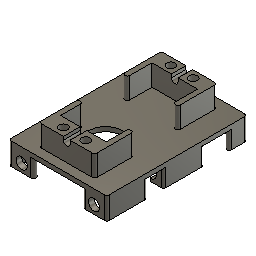
ServoMount (Autodesk Fusion 360 design; units mm, degrees)
Autodesk Fusion 360 part; units mm, degrees
note: some values were not read from the file. Set by a fixed rule: which sketch regions a step uses.
sketch "Base" plane through (0, 0, 0) normal (0, 1, 0) x (1, 0, 0)
  line L0 (0, 0) -> (44, 0)
  line L1 (44, 0) -> (44, 63)
  line L2 (44, 63) -> (0, 63)
  line L3 (0, 63) -> (0, 0)
  dimension "d1" = 44
  dimension "d2" = 63
  constraint horizontal L0
  constraint vertical L1
  constraint horizontal L2
  constraint vertical L3
  constraint coincident L0.start L3.end
  measures "d1" distance of L0.start L0.end
  measures "d2" distance of L0.start L2.end
extrude "Extrude1" add sketch "Base" along normal blind 2
sketch "Servo_Mount" plane through (0, 2, 0) normal (0, 1, 0) x (-1, 0, 0)
  line L0 (0, -63) -> (0, 0)
  line L1 (0, 0) -> (-44, 0)
  line L2 (-44, 0) -> (-44, -63)
  line L3 (-44, -63) -> (0, -63)
  line L4 (-10.75, -59) -> (-33.25, -59)
  line L5 (-33.25, -4) -> (-10.75, -4)
  line L6 (-9.5, -52.5) -> (-34.5, -52.5)
  line L7 (-9.5, -11.5) -> (-34.5, -11.5)
  line L8 (-22, 0) -> (-22, -72)
  circle A0 centre (-17, -55.75) radius 1.875
  circle A1 centre (-27, -55.75) radius 1.875
  circle A2 centre (-17, -7.5) radius 1.875
  circle A3 centre (-27, -7.5) radius 1.875
  circle A4 centre (-22, -21.5) radius 7.5
  arc A5 (-9.5, -5.25) -> (-10.75, -4) centre (-10.75, -5.25) ccw
  arc A6 (-33.25, -4) -> (-34.5, -5.25) centre (-33.25, -5.25) ccw
  arc A7 (-10.75, -59) -> (-9.5, -57.75) centre (-10.75, -57.75) ccw
  arc A8 (-34.5, -57.75) -> (-33.25, -59) centre (-33.25, -57.75) ccw
  line L9 (-11.75, -52.5) -> (-11.75, -42.625)
  line L10 (-11.75, -20.375) -> (-11.75, -11.5)
  line L11 (-9.5, -5.25) -> (-9.5, -20.375)
  line L12 (-9.5, -42.625) -> (-9.5, -57.75)
  line L13 (-32.25, -52.5) -> (-32.25, -42.625)
  line L14 (-32.25, -20.375) -> (-32.25, -11.5)
  line L15 (-34.5, -57.75) -> (-34.5, -42.625)
  line L16 (-34.5, -20.375) -> (-34.5, -5.25)
  arc A9 (-10.625, -41.5) -> (-11.75, -42.625) centre (-10.625, -42.625) ccw
  arc A10 (-9.5, -42.625) -> (-10.625, -41.5) centre (-10.625, -42.625) ccw
  arc A11 (-32.25, -42.625) -> (-33.375, -41.5) centre (-33.375, -42.625) ccw
  arc A12 (-33.375, -41.5) -> (-34.5, -42.625) centre (-33.375, -42.625) ccw
  arc A13 (-33.375, -21.5) -> (-32.25, -20.375) centre (-33.375, -20.375) ccw
  arc A14 (-34.5, -20.375) -> (-33.375, -21.5) centre (-33.375, -20.375) ccw
  arc A15 (-10.625, -21.5) -> (-9.5, -20.375) centre (-10.625, -20.375) ccw
  arc A16 (-11.75, -20.375) -> (-10.625, -21.5) centre (-10.625, -20.375) ccw
  circle A17 centre (-27, -7.5) radius 2.875
  circle A18 centre (-17, -7.5) radius 2.875
  circle A19 centre (-27, -55.75) radius 2.875
  circle A20 centre (-17, -55.75) radius 2.875
  point P0 (-9.5, -59)
  point P1 (-34.5, -59)
  point P2 (-9.5, -4)
  dimension "d5" = 25
  dimension "d6" = 55
  dimension "d7" = 4
  dimension "d8" = 9.5
  dimension "d9" = 25
  dimension "d10" = 6.5
  dimension "d11" = 7.5
  dimension "d12" = 41
  dimension "d13" = 41
  dimension "d14" = 2.25
  dimension "d15" = 2.25
  dimension "d16" = 3.75
  dimension "d17" = 3.75
  dimension "d18" = 3.25
  dimension "d19" = 3.25
  dimension "d20" = 5
  dimension "d21" = 5
  dimension "d22" = 3.75
  dimension "d23" = 3.75
  dimension "d24" = 4
  dimension "d25" = 4
  dimension "d26" = 5
  dimension "d27" = 5
  dimension "d28" = 15
  dimension "d29" = 10
  dimension "d34" = 1.25
  dimension "d35" = 1.25
  dimension "d36" = 1.25
  dimension "d37" = 1.25
  dimension "d38" = 1.125
  dimension "d39" = 1.125
  dimension "d40" = 1.125
  dimension "d41" = 1.125
  dimension "d42" = 1.125
  dimension "d43" = 1.125
  dimension "d44" = 1.125
  dimension "d45" = 1.125
  dimension "d57" = 22.25
  dimension "d119" = 5.75
  dimension "d120" = 5.75
  dimension "d121" = 5.75
  dimension "d122" = 5.75
  constraint horizontal L4
  constraint vertical L15
  constraint horizontal L5
  constraint vertical L11
  constraint coincident L6.start L11
  constraint perpendicular L6 L15
  constraint coincident L7.start L11
  constraint coincident L7.end L15
  constraint perpendicular L7 L15
  constraint coincident L6 L9.start
  constraint perpendicular L7 L9
  constraint coincident L6 L13.start
  constraint perpendicular L6 L13
  constraint midpoint L1 L8.start
  constraint perpendicular L3 L8
  constraint coincident L8 A4.centre
  constraint coincident P2 L5
  constraint coincident P2 L11
  constraint tangent L5 A5
  constraint tangent A5 L11
  constraint tangent L5 A6
  constraint tangent A6 L15
  constraint coincident P0 L4
  constraint coincident P0 L11
  constraint tangent L4 A7
  constraint tangent A7 L11
  constraint coincident P1 L15
  constraint coincident P1 L4
  constraint tangent A8 L15
  constraint tangent L4 A8
  constraint collinear L9 L10
  constraint collinear L11 L12
  constraint collinear L13 L14
  constraint collinear L15 L16
  constraint tangent L9 A9
  constraint tangent L12 A10
  constraint coincident A9.start A10.end
  constraint tangent L13 A11
  constraint tangent L15 A12
  constraint coincident A11.end A12.start
  constraint tangent L14 A13
  constraint tangent L16 A14
  constraint coincident A13.start A14.end
  constraint tangent L11 A15
  constraint tangent L10 A16
  constraint coincident A15.start A16.end
  constraint concentric A3 A17
  constraint concentric A2 A18
  constraint concentric A1 A19
  constraint concentric A0 A20
  measures "d5" distance of P0 P1
  measures "d6" distance of P0 P2
  measures "d7" distance of L3 L4
  measures "d8" distance of L0 L11
  measures "d9" distance of L6.start L6.end
  measures "d10" distance of L4 L6
  measures "d11" distance of L5 L7
  measures "d12" distance of L9.start L10.end
  measures "d13" distance of L13.start L14.end
  measures "d14" distance of L9 L11
  measures "d15" distance of L13 L15
  measures "d16" diameter of A0
  measures "d17" diameter of A1
  measures "d18" distance of L4 A0.centre
  measures "d19" distance of L4 A1.centre
  measures "d20" distance of L8 A1.centre
  measures "d21" distance of L8 A0.centre
  measures "d22" diameter of A2
  measures "d23" diameter of A3
  measures "d24" distance of L7 A3.centre
  measures "d25" distance of L7 A2.centre
  measures "d26" distance of L8 A2.centre
  measures "d27" distance of L8 A3.centre
  measures "d28" diameter of A4
  measures "d29" distance of L7 A4.centre
  measures "d34" radius of A5
  measures "d35" radius of A6
  measures "d36" radius of A7
  measures "d37" radius of A8
  measures "d38" radius of A9
  measures "d39" radius of A10
  measures "d40" radius of A11
  measures "d41" radius of A12
  measures "d42" radius of A13
  measures "d43" radius of A14
  measures "d44" radius of A15
  measures "d45" radius of A16
  measures "d57" distance of A9.centre A15.centre
  measures "d119" diameter of A17
  measures "d120" diameter of A18
  measures "d121" diameter of A19
  measures "d122" diameter of A20
extrude "Extrude2" cut sketch "Servo_Mount" against normal blind 9 contours L8 A4 | L8 A4
extrude "Extrude3" add sketch "Servo_Mount" along normal blind 9.5 contours L4 L6 L8 A7 L12 | L4 L6 L8 A8 L15 | L5 L7 L8 A6 L16 | L5 L7 L8 A5 L11 | L6 L9 L12 A9 A10 | L6 L13 L15 A11 A12 | L7 L10 L11 A15 A16 | L7 L14 L16 A13 A14 | A17 | A18 | A19 | A20
sketch "Top_Through_Front" plane through (0, 0, -4) normal (0, 0, 1) x (1, 0, 0)
  line L0 (10.75, 2) -> (33.25, 2)
  line L1 (33.25, 2) -> (33.25, 11.5)
  line L2 (33.25, 11.5) -> (10.75, 11.5)
  line L3 (10.75, 11.5) -> (10.75, 2)
  line L4 (20.5, 11.5) -> (23.5, 11.5)
  line L5 (23.5, 11.5) -> (23.5, 10)
  line L6 (20.5, 10) -> (20.5, 11.5)
  arc A0 (20.5, 10) -> (22, 8.5) centre (22, 10) ccw
  arc A1 (22, 8.5) -> (23.5, 10) centre (22, 10) ccw
  point P0 (20.5, 8.5)
  dimension "d50" = 3
  dimension "d51" = 3
  dimension "d52" = 9.75
  dimension "d53" = 1.5
  dimension "d54" = 1.5
  constraint horizontal L4
  constraint vertical L5
  constraint vertical L6
  constraint coincident L2 L4.start
  constraint coincident P0 L6
  constraint tangent L6 A0
  constraint tangent L5 A1
  constraint coincident A0.end A1.start
  measures "d50" distance of L4.start L4.end
  measures "d51" distance of L4.start P0
  measures "d52" distance of L1 L5
  measures "d53" radius of A0
  measures "d54" radius of A1
extrude "Extrude4" cut sketch "Top_Through_Front" against normal blind 15 contours L2 L4 L5 L6 A0 A1
sketch "Top_Through_Back" plane through (0, 0, -59) normal (0, 0, -1) x (-1, 0, 0)
  line L0 (-33.25, 2) -> (-10.75, 2)
  line L1 (-10.75, 2) -> (-10.75, 11.5)
  line L2 (-10.75, 11.5) -> (-33.25, 11.5)
  line L3 (-33.25, 11.5) -> (-33.25, 2)
  line L4 (-23.5, 11.5) -> (-20.5, 11.5)
  line L5 (-20.5, 11.5) -> (-20.5, 10)
  line L6 (-23.5, 10) -> (-23.5, 11.5)
  arc A0 (-22, 8.5) -> (-20.5, 10) centre (-22, 10) ccw
  arc A1 (-23.5, 10) -> (-22, 8.5) centre (-22, 10) ccw
  point P0 (-23.5, 8.5)
  dimension "d58" = 3
  dimension "d59" = 3
  dimension "d60" = 9.75
  dimension "d61" = 1.5
  dimension "d62" = 1.5
  constraint horizontal L4
  constraint vertical L5
  constraint vertical L6
  constraint coincident L2 L4.start
  constraint tangent L5 A0
  constraint coincident P0 L6
  constraint tangent L6 A1
  constraint coincident A0.start A1.end
  measures "d58" distance of L4.start L4.end
  measures "d59" distance of L4.start P0
  measures "d60" distance of L1 L5
  measures "d61" radius of A0
  measures "d62" radius of A1
extrude "Extrude5" cut sketch "Top_Through_Back" against normal blind 13 contours L2 L4 L5 L6 A0 A1
sketch "Back_Side" plane through (0, 0, 0) normal (0, -1, 0) x (1, 0, 0)
  circle A0 centre (22, -21.5) radius 7.5
  line L0 (0, 0) -> (0, -63)
  line L1 (0, -63) -> (44, -63)
  line L2 (44, -63) -> (44, 0)
  line L3 (44, 0) -> (0, 0)
  line L4 (1, -63) -> (10, -63)
  line L5 (10, -61) -> (3, -61)
  line L6 (0, -61) -> (0, -62)
  arc A1 (10, -63) -> (11, -62) centre (10, -62) ccw
  arc A2 (11, -62) -> (10, -61) centre (10, -62) ccw
  arc A3 (0, -62) -> (1, -63) centre (1, -62) ccw
  line L7 (1, -63) -> (2, -63)
  line L8 (2, -60) -> (2, -56)
  line L9 (0, -56) -> (0, -62)
  arc A4 (2, -60) -> (3, -61) centre (3, -60) ccw
  arc A5 (2, -56) -> (1, -55) centre (1, -56) ccw
  arc A6 (1, -55) -> (0, -56) centre (1, -56) ccw
  line L10 (1, -43.5) -> (9.75, -43.5)
  line L11 (9.75, -41) -> (2.5, -41)
  line L12 (0, -41) -> (0, -42.5)
  arc A7 (9.75, -43.5) -> (11, -42.25) centre (9.75, -42.25) ccw
  arc A8 (11, -42.25) -> (9.75, -41) centre (9.75, -42.25) ccw
  line L13 (2.5, -41) -> (2.5, -33.5)
  line L14 (0, -26.5) -> (0, -41)
  arc A9 (0, -42.5) -> (1, -43.5) centre (1, -42.5) ccw
  arc A10 (1, -25.5) -> (0, -26.5) centre (1, -26.5) ccw
  line L15 (1, 0) -> (9.75, 0)
  line L16 (9.75, -2.5) -> (2.5, -2.5)
  line L17 (0, -2.5) -> (0, -1)
  arc A11 (11, -1.25) -> (9.75, 0) centre (9.75, -1.25) ccw
  arc A12 (9.75, -2.5) -> (11, -1.25) centre (9.75, -1.25) ccw
  arc A13 (1, 0) -> (0, -1) centre (1, -1) ccw
  line L18 (2.5, -2.5) -> (2.5, -9.5)
  line L19 (0, -17) -> (0, -2.5)
  arc A14 (0, -17) -> (1, -18) centre (1, -17) ccw
  line L20 (43, -63) -> (34, -63)
  line L21 (34, -61) -> (41, -61)
  line L22 (44, -61) -> (44, -62)
  arc A15 (33, -62) -> (34, -63) centre (34, -62) ccw
  arc A16 (34, -61) -> (33, -62) centre (34, -62) ccw
  line L23 (43, -63) -> (42, -63)
  line L24 (42, -60) -> (42, -56)
  line L25 (44, -56) -> (44, -62)
  arc A17 (43, -55) -> (42, -56) centre (43, -56) ccw
  arc A18 (44, -56) -> (43, -55) centre (43, -56) ccw
  arc A19 (41, -61) -> (42, -60) centre (41, -60) ccw
  arc A20 (43, -63) -> (44, -62) centre (43, -62) ccw
  line L26 (43, -43.5) -> (34.25, -43.5)
  line L27 (34.25, -41) -> (41.5, -41)
  line L28 (44, -41) -> (44, -42.5)
  line L29 (41.5, -41) -> (41.5, -33.5)
  line L30 (41.5, -25.5) -> (43, -25.5)
  line L31 (44, -26.5) -> (44, -41)
  arc A21 (33, -42.25) -> (34.25, -43.5) centre (34.25, -42.25) ccw
  arc A22 (34.25, -41) -> (33, -42.25) centre (34.25, -42.25) ccw
  arc A23 (43, -43.5) -> (44, -42.5) centre (43, -42.5) ccw
  arc A24 (44, -26.5) -> (43, -25.5) centre (43, -26.5) ccw
  line L32 (43, 0) -> (34.25, 0)
  line L33 (34.25, -2.5) -> (41.5, -2.5)
  line L34 (44, -2.5) -> (44, -1)
  line L35 (41.5, -2.5) -> (41.5, -9.5)
  line L36 (44, -17) -> (44, -2.5)
  arc A25 (33, -1.25) -> (34.25, -2.5) centre (34.25, -1.25) ccw
  arc A26 (34.25, 0) -> (33, -1.25) centre (34.25, -1.25) ccw
  arc A27 (44, -1) -> (43, 0) centre (43, -1) ccw
  arc A28 (43, -18) -> (44, -17) centre (43, -17) ccw
  line L37 (43, -25.5) -> (38, -25.5)
  line L38 (38, -25.5) -> (38, -32.5)
  line L39 (38, -32.5) -> (40.5, -32.5)
  arc A29 (41.5, -33.5) -> (40.5, -32.5) centre (40.5, -33.5) ccw
  line L40 (1, -25.5) -> (6, -25.5)
  line L41 (6, -25.5) -> (6, -32.5)
  line L42 (6, -32.5) -> (3.5, -32.5)
  arc A30 (3.5, -32.5) -> (2.5, -33.5) centre (3.5, -33.5) ccw
  line L43 (43, -18) -> (38, -18)
  line L44 (38, -18) -> (38, -10.5)
  line L45 (38, -10.5) -> (40.5, -10.5)
  arc A31 (40.5, -10.5) -> (41.5, -9.5) centre (40.5, -9.5) ccw
  line L46 (1, -18) -> (6, -18)
  line L47 (6, -18) -> (6, -10.5)
  line L48 (6, -10.5) -> (3.5, -10.5)
  arc A32 (2.5, -9.5) -> (3.5, -10.5) centre (3.5, -9.5) ccw
  point P0 (0, -63)
  point P1 (11, -63)
  point P2 (0, -55)
  point P3 (0, -43.5)
  point P4 (11, -43.5)
  point P5 (0, -25.5)
  point P6 (11, 0)
  point P7 (0, -18)
  point P8 (33, -63)
  point P9 (44, -55)
  point P10 (44, -43.5)
  point P11 (33, -43.5)
  point P12 (44, -25.5)
  point P13 (44, 0)
  point P14 (33, 0)
  point P15 (44, -18)
  dimension "d65" = 11
  dimension "d66" = 2
  dimension "d67" = 1
  dimension "d68" = 1
  dimension "d69" = 1
  dimension "d70" = 2
  dimension "d71" = 8
  dimension "d72" = 1
  dimension "d73" = 1
  dimension "d74" = 1
  dimension "d75" = 11
  dimension "d76" = 2.5
  dimension "d77" = 17.5
  dimension "d78" = 1.25
  dimension "d79" = 1.25
  dimension "d80" = 2.5
  dimension "d81" = 15.5
  dimension "d82" = 1
  dimension "d83" = 1
  dimension "d84" = 11
  dimension "d85" = 2.5
  dimension "d86" = 1.25
  dimension "d87" = 1.25
  dimension "d88" = 1
  dimension "d89" = 2.5
  dimension "d90" = 15.5
  dimension "d91" = 1
  dimension "d92" = 11
  dimension "d93" = 2
  dimension "d94" = 1
  dimension "d95" = 1
  dimension "d96" = 2
  dimension "d97" = 8
  dimension "d98" = 1
  dimension "d99" = 1
  dimension "d100" = 1
  dimension "d101" = 1
  dimension "d102" = 11
  dimension "d103" = 2.5
  dimension "d104" = 17.5
  dimension "d105" = 2.5
  dimension "d106" = 15.5
  dimension "d107" = 1.25
  dimension "d108" = 1.25
  dimension "d109" = 1
  dimension "d110" = 1
  dimension "d111" = 11
  dimension "d112" = 2.5
  dimension "d113" = 2.5
  dimension "d114" = 15.5
  dimension "d115" = 1.25
  dimension "d116" = 1.25
  dimension "d117" = 1
  dimension "d118" = 1
  dimension "d125" = 6
  dimension "d127" = 1
  dimension "d129" = 6
  dimension "d131" = 1
  dimension "d132" = 7
  dimension "d133" = 7
  dimension "d135" = 6
  dimension "d137" = 1
  dimension "d138" = 7.5
  dimension "d139" = 6
  dimension "d141" = 1
  dimension "d142" = 7.5
  dimension "d144" = 8
  dimension "d145" = 8
  dimension "d146" = 8.5
  dimension "d147" = 8.5
  constraint horizontal L4
  constraint horizontal L5
  constraint vertical L6
  constraint coincident P0 L0.end
  constraint coincident P1 L4
  constraint tangent L4 A1
  constraint tangent L5 A2
  constraint coincident A1.end A2.start
  constraint coincident P0 L4
  constraint coincident P0 L6
  constraint tangent L4 A3
  constraint tangent L6 A3
  constraint horizontal L7
  constraint vertical L8
  constraint vertical L9
  constraint coincident L6.start L5
  constraint coincident L7.end L8
  constraint tangent L5 A4
  constraint tangent L8 A4
  constraint tangent L8 A5
  constraint coincident P2 L9
  constraint tangent L9 A6
  constraint coincident A5.end A6.start
  constraint horizontal L10
  constraint horizontal L11
  constraint vertical L12
  constraint coincident L0 P3
  constraint coincident P4 L10
  constraint tangent L10 A7
  constraint tangent L11 A8
  constraint coincident A7.end A8.start
  constraint vertical L13
  constraint vertical L14
  constraint coincident P3 L10
  constraint coincident P3 L12
  constraint tangent L10 A9
  constraint tangent L12 A9
  constraint coincident P5 L14
  constraint tangent L14 A10
  constraint horizontal L15
  constraint horizontal L16
  constraint vertical L17
  constraint coincident L0.start L3.end
  constraint coincident P6 L15
  constraint tangent L15 A11
  constraint tangent L16 A12
  constraint coincident A11.start A12.end
  constraint coincident L0.start L15
  constraint coincident L0.start L17
  constraint tangent L15 A13
  constraint tangent L17 A13
  constraint vertical L18
  constraint vertical L19
  constraint coincident P7 L19
  constraint tangent L19 A14
  constraint horizontal L20
  constraint horizontal L21
  constraint vertical L22
  constraint coincident P8 L20
  constraint tangent L20 A15
  constraint tangent L21 A16
  constraint coincident A15.start A16.end
  constraint horizontal L23
  constraint vertical L24
  constraint vertical L25
  constraint tangent L24 A17
  constraint coincident P9 L25
  constraint tangent L25 A18
  constraint coincident A17.start A18.end
  constraint coincident L22.start L21
  constraint coincident L23.end L24
  constraint tangent L21 A19
  constraint tangent L24 A19
  constraint tangent L23 A20
  constraint tangent L25 A20
  constraint horizontal L26
  constraint horizontal L27
  constraint vertical L28
  constraint coincident L2 P10
  constraint vertical L29
  constraint horizontal L30
  constraint vertical L31
  constraint coincident P11 L26
  constraint tangent L26 A21
  constraint tangent L27 A22
  constraint coincident A21.start A22.end
  constraint coincident P10 L26
  constraint coincident P10 L28
  constraint tangent L26 A23
  constraint tangent L28 A23
  constraint coincident P12 L31
  constraint coincident P12 L30
  constraint tangent L31 A24
  constraint tangent L30 A24
  constraint horizontal L32
  constraint horizontal L33
  constraint vertical L34
  constraint coincident P13 L2.end
  constraint vertical L35
  constraint vertical L36
  constraint tangent L33 A25
  constraint coincident P14 L32
  constraint tangent L32 A26
  constraint coincident A25.start A26.end
  constraint coincident P13 L34
  constraint coincident P13 L32
  constraint tangent L34 A27
  constraint tangent L32 A27
  constraint coincident P15 L36
  constraint tangent L36 A28
  constraint horizontal L37
  constraint vertical L38
  constraint horizontal L39
  constraint tangent L29 A29
  constraint tangent L39 A29
  constraint horizontal L40
  constraint vertical L41
  constraint horizontal L42
  constraint tangent L13 A30
  constraint tangent L42 A30
  constraint horizontal L43
  constraint vertical L44
  constraint horizontal L45
  constraint tangent L45 A31
  constraint tangent L35 A31
  constraint horizontal L46
  constraint vertical L47
  constraint horizontal L48
  constraint tangent L48 A32
  constraint tangent L18 A32
  measures "d65" distance of P0 P1
  measures "d66" distance of P0 L6.start
  measures "d67" radius of A1
  measures "d68" radius of A2
  measures "d69" radius of A3
  measures "d70" distance of P0 L7.end
  measures "d71" distance of P0 P2
  measures "d72" radius of A4
  measures "d73" radius of A5
  measures "d74" radius of A6
  measures "d75" distance of P3 P4
  measures "d76" distance of P3 L12.start
  measures "d77" distance of L5 L10
  measures "d78" radius of A7
  measures "d79" radius of A8
  measures "d80" distance of L12.start L11.end
  measures "d81" distance of L12.start P5
  measures "d82" radius of A9
  measures "d83" radius of A10
  measures "d84" distance of L0.start P6
  measures "d85" distance of L0.start L17.start
  measures "d86" radius of A11
  measures "d87" radius of A12
  measures "d88" radius of A13
  measures "d89" distance of L17.start L16.end
  measures "d90" distance of L17.start P7
  measures "d91" radius of A14
  measures "d92" distance of L1.end P8
  measures "d93" distance of L1.end L22.start
  measures "d94" radius of A15
  measures "d95" radius of A16
  measures "d96" distance of L1.end L23.end
  measures "d97" distance of L1.end P9
  measures "d98" radius of A17
  measures "d99" radius of A18
  measures "d100" radius of A19
  measures "d101" radius of A20
  measures "d102" distance of P10 P11
  measures "d103" distance of P10 L28.start
  measures "d104" distance of L21 L26
  measures "d105" distance of L28.start L27.end
  measures "d106" distance of L28.start P12
  measures "d107" radius of A21
  measures "d108" radius of A22
  measures "d109" radius of A23
  measures "d110" radius of A24
  measures "d111" distance of P13 P14
  measures "d112" distance of P13 L34.start
  measures "d113" distance of L34.start L33.end
  measures "d114" distance of L34.start P15
  measures "d115" radius of A25
  measures "d116" radius of A26
  measures "d117" radius of A27
  measures "d118" radius of A28
  measures "d125" distance of P12 L37.end
  measures "d127" radius of A29
  measures "d129" distance of P5 L40.end
  measures "d131" radius of A30
  measures "d132" distance of L37.end L38.end
  measures "d133" distance of L40.end L41.end
  measures "d135" distance of P15 L43.end
  measures "d137" radius of A31
  measures "d138" distance of L43.end L44.end
  measures "d139" distance of P7 L46.end
  measures "d141" radius of A32
  measures "d142" distance of L46.end L47.end
  measures "d144" distance of L16 L48
  measures "d145" distance of L33 L45
  measures "d146" distance of L27 L39
  measures "d147" distance of L11 L42
extrude "Extrude6" cut sketch "Servo_Mount" against normal blind 8 contours A0 | A1 | A2 | A3 | A17 | A18 | A19 | A20
extrude "Extrude7" add sketch "Back_Side" along normal blind 8 contours L0 L3 L15 L16 L17 A11 A12 A13 L18 L19 A14 L46 L47 L48 A32 | L2 L3 L32 L33 L34 L35 L36 A25 A26 A27 A28 L43 L44 L45 A31 | L0 L10 L11 L12 A7 A8 L13 L14 A9 A10 L40 L41 L42 A30 | L0 L1 L4 L5 L6 A1 A2 A3 L7 L8 L9 A4 A5 A6 | L2 L26 L27 L28 L29 L30 L31 A21 A22 A23 A24 L37 L38 L39 A29 | L1 L2 L20 L21 L22 A15 A16 L23 L24 L25 A17 A18 A19 A20
fillet "Fillet1" radius 1 1 edges at (0, 1, 0)
fillet "Fillet2" radius 1 1 edges at (0, 1, -63)
fillet "Fillet3" radius 1 1 edges at (44, 1, -63)
fillet "Fillet4" radius 1 1 edges at (44, 1, 0)
sketch "Through_Holes_Tube" plane through (0, 0, 0) normal (0, 0, 1) x (1, 0, 0)
  line L0 (43, -8) -> (43, 2)
  line L1 (43, 2) -> (1, 2)
  line L2 (1, 2) -> (1, -8)
  line L3 (1, -8) -> (9.75, -8)
  line L4 (9.75, -8) -> (9.75, 0)
  line L5 (9.75, 0) -> (34.25, 0)
  line L6 (34.25, 0) -> (34.25, -8)
  line L7 (34.25, -8) -> (43, -8)
  circle A0 centre (38.25, -4.25) radius 2.5
  circle A1 centre (5.75, -4.25) radius 2.5
  dimension "d158" = 5
  dimension "d159" = 4
  dimension "d161" = 3.75
  dimension "d162" = 5
  dimension "d163" = 3.75
  dimension "d164" = 4
  measures "d158" diameter of A0
  measures "d159" distance of L6 A0.centre
  measures "d161" distance of L7 A0.centre
  measures "d162" diameter of A1
  measures "d163" distance of L3 A1.centre
  measures "d164" distance of L4 A1.centre
extrude "Extrude8" cut sketch "Through_Holes_Tube" against normal blind 76 contours A0 | A1
